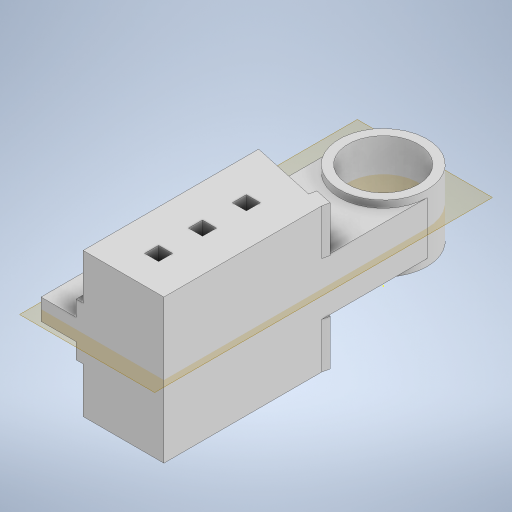
# Autodesk Inventor part: Part10copycopy
Saved by Autodesk Inventor 2023 (Build 270158000, 158)
## iProperties
Created: 2024-11-26
Part Number: Part10copycopy
Material: Generic
Document SubType Name: Modeling
Designer: 1ZHUSAM
Density: 1 g/cm^3
Appearance: Default
Author: 1ZHUSAM
Autodesk Inventor part; units mm, degrees
ref_plane "YZ Plane" through (0, 0, 0) normal (1, 0, 0) x (0, 1, 0)
ref_plane "XY Plane" through (0, 0, 0) normal (0, 0, 1) x (1, 0, 0)
sketch "Sketch1" plane through (0, 0, 0) normal (0, 1, 0) x (-1, 0, 0)
  circle A0 centre (0, 0) radius 10
  circle A1 centre (0, 0) radius 12.5
  line L0 (12.5, 0) -> (12.5, 50)
  line L1 (-12.5, 0) -> (-12.5, 50)
  line L2 (-12.5, 50) -> (12.5, 50)
  dimension "d0" = 20
  dimension "d1" = 25
  dimension "d2" = 50
  constraints: 6 end point, 2 centre point, 2 coincident, 2 point on circle, 2 tangent, 2 vertical, 1 perpendicular
  measures "d0" diameter of A0
  measures "d1" diameter of A1
  measures "d2" distance of L0.start L0.end
extrude "Extrusion1" add sketch "Sketch1" along normal blind 15
sketch "Sketch2" plane through (-12.5, 0, 0) normal (-1, 0, 0) x (0, 0, 1)
  line L0 (-12.5, 0) -> (-12.5, 15) projected
  line L1 (-12.5, 7.5) -> (37.5, 7.5)
  line L2 (25, 7.5) -> (25, 4.5)
  line L3 (25, 4.5) -> (25, 10.5)
  line L4 (25, 10.5) -> (75, 10.5)
  line L5 (75, 10.5) -> (75, 4.5)
  line L6 (75, 4.5) -> (25, 4.5)
  point P0 (0, 0)
  dimension "d5" = 50
  dimension "d8" = 3
  dimension "d9" = 6
  dimension "d10" = 50
  constraints: 12 end point, 3 perpendicular, 2 horizontal, 2 point on line, 1 midpoint
  measures "d5" distance of L1.start L1.end
  measures "d8" distance of L2.start L2.end
  measures "d9" distance of L2.end L3.end
  measures "d10" distance of L3.end L4.end
extrude "Extrusion2" add sketch "Sketch2" along normal blind 10
sketch "Sketch3" plane through (-12.5, 0, 50) normal (0, 0, 1) x (1, 0, 0)
  point P0 (12.5, 0)
sketch "Sketch4" plane through (-12.5, 0, 50) normal (0, 0, 1) x (1, 0, 0)
  line L0 (25, 0) -> (25, 15) projected
  line L1 (25, 0) -> (25, 15)
  line L2 (0, 15) -> (25, 15) projected
  line L3 (25, 15) -> (0, 15)
  line L4 (0, 0) -> (0, 15) projected
  line L5 (0, 15) -> (0, 0)
  line L6 (0, 0) -> (25, 0) projected
  line L7 (0, 0) -> (25, 0)
  point P0 (12.5, 0)
  constraints: 8 end point, 4 collinear
extrude "Extrusion3" add sketch "Sketch4" along normal blind 25
sketch "Sketch5" plane through (-12.5, 4.5, 25) normal (0, -1, 0) x (1, 0, 0)
  point P0 (12.5, -25)
sketch "Sketch8" plane through (-12.5, 4.5, 25) normal (0, -1, 0) x (1, 0, 0)
  line L0 (0, 0) -> (-10, 0) projected
  line L1 (-5, 0) -> (-5, 50)
  line L2 (0, 50) -> (-10, 50) projected
  line L3 (-3, 12) -> (-7, 12)
  line L4 (-7, 12) -> (-7, 8)
  line L5 (-7, 8) -> (-3, 8)
  line L6 (-3, 8) -> (-3, 12)
  line L7 (-3, 12) -> (-7, 8) construction
  line L8 (-7, 12) -> (-3, 8) construction
  line L9 (-5, 10) -> (-5, 23)
  line L10 (-7, 21) -> (-3, 21)
  line L11 (-3, 21) -> (-3, 25)
  line L12 (-3, 25) -> (-7, 25)
  line L13 (-7, 25) -> (-7, 21)
  line L14 (-7, 21) -> (-3, 25) construction
  line L15 (-3, 21) -> (-7, 25) construction
  line L16 (-5, 23) -> (-5, 36)
  line L17 (-7, 34) -> (-3, 34)
  line L18 (-3, 34) -> (-3, 38)
  line L19 (-3, 38) -> (-7, 38)
  line L20 (-7, 38) -> (-7, 34)
  line L21 (-7, 34) -> (-3, 38) construction
  line L22 (-3, 34) -> (-7, 38) construction
  point P0 (12.5, -25)
  dimension "d40" = 4
  dimension "d41" = 4
  dimension "d42" = 13
  dimension "d43" = 4
  dimension "d44" = 4
  dimension "d45" = 13
  dimension "d46" = 4
  dimension "d47" = 4
  constraints: 42 end point, 8 midpoint, 6 parallel, 3 horizontal, 3 perpendicular, 3 point on line
  measures "d40" distance of L5.end L4.end
  measures "d41" distance of L4.end L3.end
  measures "d42" distance of L9.start L9.end
  measures "d43" distance of L12.end L11.end
  measures "d44" distance of L11.end L10.end
  measures "d45" distance of L9.end L16.end
  measures "d46" distance of L19.end L18.end
  measures "d47" distance of L18.end L17.end
extrude "Extrusion6" cut sketch "Sketch8" against normal blind 10
sketch "Sketch9" plane through (0, 0, 0) normal (0, -1, 0) x (1, 0, 0)
  line L0 (-12.5, 25) -> (-22.5, 25) projected
  line L1 (-12.5, 25) -> (12.5, 25)
  line L2 (12.5, 0) -> (12.5, 75) projected
  line L3 (-12.5, 25) -> (-12.5, 75) projected
  line L4 (-12.5, 25) -> (-12.5, 75)
  line L5 (-12.5, 75) -> (12.5, 75) projected
  line L6 (-12.5, 75) -> (12.5, 75)
  line L7 (12.5, 75) -> (12.5, 25)
  line L8 (12.5, 0) -> (12.5, 30)
  line L9 (-12.5, 25) -> (-10.5, 25)
  line L10 (-10.5, 25) -> (-10.5, 75)
  line L11 (-12.5, 75) -> (-12.5, 25)
  line L12 (-10.5, 25) -> (12.5, 30)
  point P0 (0, 0)
  dimension "d50" = 30
  dimension "d51" = 2
  constraints: 18 end point, 5 point on line, 3 collinear, 2 perpendicular, 1 horizontal
  measures "d50" distance of L8.start L8.end
  measures "d51" distance of L0.start L9.end
extrude "Extrusion7" add sketch "Sketch9" along normal blind 13 contours L10 L5 L2 L12
sketch "Sketch10" plane through (0, -13, 0) normal (0, -1, 0) x (1, 0, 0)
  point P0 (0, 0)
sketch "Sketch11" plane through (0, -13, 0) normal (0, -1, 0) x (1, 0, 0)
  line L0 (-10.5, 25) -> (12.5, 30) projected
  line L1 (12.5, 30) -> (-10.5, 30)
  line L2 (-10.5, 25) -> (-10.5, 75) projected
  line L3 (-10.5, 30) -> (1, 30)
  line L4 (1, 30) -> (1, 75)
  line L5 (12.5, 75) -> (-12.5, 75) projected
  line L6 (-1, 42) -> (3, 42)
  line L7 (3, 42) -> (3, 38)
  line L8 (3, 38) -> (-1, 38)
  line L9 (-1, 38) -> (-1, 42)
  line L10 (-1, 42) -> (3, 38) construction
  line L11 (3, 42) -> (-1, 38) construction
  line L12 (1, 40) -> (1, 52.5)
  line L13 (-1, 50.5) -> (3, 50.5)
  line L14 (3, 50.5) -> (3, 54.5)
  line L15 (3, 54.5) -> (-1, 54.5)
  line L16 (-1, 54.5) -> (-1, 50.5)
  line L17 (-1, 50.5) -> (3, 54.5) construction
  line L18 (3, 50.5) -> (-1, 54.5) construction
  line L19 (1, 52.5) -> (1, 65)
  line L20 (-1, 63) -> (3, 63)
  line L21 (3, 63) -> (3, 67)
  line L22 (3, 67) -> (-1, 67)
  line L23 (-1, 67) -> (-1, 63)
  line L24 (-1, 63) -> (3, 67) construction
  line L25 (3, 63) -> (-1, 67) construction
  line L26 (-1, 38) -> (-1, 42)
  line L27 (-1, 38) -> (3, 38)
  line L28 (3, 38) -> (3, 42)
  line L29 (3, 42) -> (-1, 42)
  line L30 (-1, 42) -> (-1, 38)
  line L31 (-1, 38) -> (3, 42) construction
  line L32 (3, 38) -> (-1, 42) construction
  point P0 (0, 0)
  dimension "d54" = 11.5
  dimension "d55" = 4
  dimension "d56" = 4
  dimension "d57" = 12.5
  dimension "d58" = 4
  dimension "d59" = 4
  dimension "d60" = 12.5
  dimension "d61" = 4
  dimension "d62" = 4
  constraints: 60 end point, 10 midpoint, 9 equal length, 5 horizontal, 5 perpendicular, 4 point on line
  measures "d54" distance of L1.end L3.end
  measures "d55" distance of L7.end L8.end
  measures "d56" distance of L6.end L7.end
  measures "d57" distance of L12.start L12.end
  measures "d58" distance of L15.end L14.end
  measures "d59" distance of L14.end L13.end
  measures "d60" distance of L12.end L19.end
  measures "d61" distance of L22.end L21.end
  measures "d62" distance of L21.end L20.end
extrude "Extrusion8" cut sketch "Sketch11" against normal blind 50 contours L8 L9 L6 L4 | L4 L6 L7 L8 | L22 L21 L20 L4 | L4 L20 L23 L22 | L13 L16 L15 L4 | L4 L15 L14 L13
ref_plane "Work Plane1" through (0, 7.5, 0) normal (0, 1, 0) x (-1, 0, 0)
mirror "Mirror1" about plane through (0, 7.5, 0) normal (0, 1, 0) of "Extrusion7"
mirror "Mirror2" about plane through (0, 7.5, 0) normal (0, 1, 0) of "Extrusion8"
sketch "Sketch12" plane through (-22.5, 0, 0) normal (-1, 0, 0) x (0, 0, 1)
  point P0 (0, 0)
sketch "Sketch13" plane through (-12.5, 4.5, 25) normal (0, -1, 0) x (1, 0, 0)
  point P0 (12.5, -25)
sketch "Sketch14" plane through (-12.5, 4.5, 25) normal (0, -1, 0) x (1, 0, 0)
  point P0 (12.5, -25)
sketch "Sketch15" plane through (-10.5, 15, 25) normal (0.2124296, 0, -0.9771764) x (-0.9771764, 0, -0.2124296)
  line L0 (-23.5372, 0) -> (-23.5372, 13) projected
  line L1 (-14.7001, 13) -> (-18.6088, 13) projected
  line L2 (-23.5372, 0) -> (-18.5372, 0)
  line L3 (-18.5372, 0) -> (-18.5372, 13)
  line L4 (-18.5372, 13) -> (-23.5372, 13)
  line L5 (-23.5372, 13) -> (-23.5372, 0)
  line L6 (-23.5372, -28) -> (-33.0965, -28) projected
  line L7 (-18.6088, -28) -> (-18.6088, 13) projected
  line L8 (-23.5372, -28) -> (-18.6088, -28)
  line L9 (-18.6088, -28) -> (-18.6088, -15)
  line L10 (-18.6088, -15) -> (-23.5372, -15)
  line L11 (-23.5372, -15) -> (-23.5372, -28)
  point P0 (-4.9496, -15)
  point P1 (-18.6088, 0)
  dimension "d66" = 5
  constraints: 16 end point, 4 parallel, 2 horizontal, 2 perpendicular, 2 point on line
  measures "d66" distance of L4.end L3.end
extrude "Extrusion9" add sketch "Sketch15" along normal blind 2 contours L0 L4 L7 L2 | L8 L11 L10 L7
sketch "Sketch16" plane through (0, 15, 0) normal (0, 1, 0) x (1, 0, 0)
  circle A0 centre (0, 0) radius 10
  circle A1 centre (0, 0) radius 12.5
  dimension "d69" = 25
  constraints: 2 centre point, 2 coincident
  measures "d69" diameter of A1
extrude "Extrusion10" add sketch "Sketch16" along normal blind 2
sketch "Sketch17" plane through (0, 0, 0) normal (0, -1, 0) x (1, 0, 0)
  circle A0 centre (0, 0) radius 10
  circle A1 centre (0, 0) radius 10 projected
  circle A2 centre (0, 0) radius 12.5
  constraints: 2 centre point, 2 coincident
extrude "Extrusion11" add sketch "Sketch17" along normal blind 2
body "Solid1"
